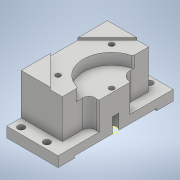
# Autodesk Inventor part: FAB-OX0001
Saved by Autodesk Inventor 2020 (Build 240168000, 168)
## iProperties
Created: 2017-01-19
Part Number: FAB-OX0001
Material: Generic
Document SubType Name: Modeling
Designer: map
Density: 1 g/cm^3
Appearance: Default
Author: map
Revision Number: 01
Autodesk Inventor part; units mm, degrees
ref_plane "YZ Plane" through (0, 0, 0) normal (1, 0, 0) x (0, 1, 0)
ref_plane "XZ Plane" through (0, 0, 0) normal (0, 1, 0) x (-1, 0, 0)
derived "FAB-P0038 - BS2 Optics Mount.ipt"
sketch "EXPORTED" plane through (-45, 40, 0) normal (0, 0, -1) x (-1, 0, 0)
  circle A0 centre (-33, -90) radius 3.3
  circle A1 centre (-8, -90) radius 3.3
  circle A2 centre (-19.9813, -66.0965) radius 4
  circle A3 centre (-46.0778, -40) radius 4
  circle A4 centre (-19.9813, -13.9035) radius 4
  circle A5 centre (-33, 10) radius 3.3
  circle A6 centre (-8, 10) radius 3.3
  circle A7 centre (-20.5, 10) radius 2
  line L0 (-5.7006, -21) -> (-19.7006, -7)
  line L1 (-19.7006, -73) -> (-5.7006, -59)
  line L2 (0, -97) -> (-50.5, -97)
  line L3 (-50.5, -97) -> (-50.5, -80)
  line L4 (0, -80) -> (0, -97)
  line L5 (0, 17) -> (0, 0)
  line L6 (-50.5, 17) -> (0, 17)
  line L7 (-50.5, 0) -> (-50.5, 17)
  point P0 (-45, -40)
ref_plane "LensMountFoot" through (-25.2994, 33, 47.902) normal (0, 0, 1) x (1, 0, 0)
ref_plane "GoniometerFoot" through (-11, -6, 37) normal (0, 0, 1) x (1, 0, 0)
ref_plane "Table" through (-45, 40, 0) normal (0, 0, -1) x (-1, 0, 0)
sketch "Sketch8" plane through (-45, 40, 0) normal (0, 0, -1) x (-1, 0, 0)
  line L0 (0, -96) -> (-50.5, -96)
  line L1 (-50.5, -96) -> (-50.5, 16)
  line L2 (-50.5, 16) -> (0, 16)
  line L3 (0, 16) -> (0, -96)
  line L4 (0, -80) -> (0, -97) projected
  line L5 (-50.5, -97) -> (-50.5, -80) projected
  circle A0 centre (-8, -90) radius 3.3 construction
  circle A1 centre (-8, 10) radius 3.3 construction
  line L6 (0, -40) -> (-50.5, -40) construction
  line L7 (-8, -90) -> (-8, 10) construction
  point P0 (-45, -40)
  point P1 (-8, -40)
  dimension "d15" = 112
  constraints: 12 end point, 3 midpoint, 2 collinear, 2 parallel, 1 horizontal, 1 perpendicular, 1 point on line, 1 vertical
  measures "d15" distance of L0.end L1.end
extrude "Bulk" add sketch "Sketch8" against normal up to surface (47.902 mm away)
ref_plane "Work Plane7" through (-45, 40, 10) normal (0, 0, -1) x (-1, 0, 0)
sketch "Sketch11" plane through (-45, 40, 10) normal (0, 0, -1) x (-1, 0, 0)
  circle A0 centre (-33, -90) radius 3.3 construction
  circle A1 centre (-8, -90) radius 3.3 construction
  circle A2 centre (-33, 10) radius 3.3 construction
  circle A3 centre (-8, 10) radius 3.3 construction
  line L0 (-50.5, -96) -> (-50.5, 16) construction
  line L1 (0, 16) -> (0, -96) construction
  line L2 (-50.5, -96) -> (0, -96)
  line L3 (0, -96) -> (0, -82)
  line L4 (0, -82) -> (-50.5, -82)
  line L5 (-50.5, -82) -> (-50.5, -96)
  line L6 (-50.5, 2) -> (0, 2)
  line L7 (0, 2) -> (0, 16)
  line L8 (0, 16) -> (-50.5, 16)
  line L9 (-50.5, 16) -> (-50.5, 2)
  line L10 (-50.5, -96) -> (0, -96) construction
  point P0 (-45, -40)
  point P1 (0, -89)
  dimension "d38" = 8
  constraints: 16 end point, 4 parallel, 3 point on line, 2 horizontal, 2 perpendicular, 1 collinear, 1 midpoint
  measures "d38" distance from line of L4 A0.centre
extrude "Feet" cut sketch "Sketch11" against normal through all
sketch "AlignmentFeatures" plane through (-45, 40, 0) normal (0, 0, -1) x (-1, 0, 0)
  line L0 (-19.9813, 10) -> (-19.9813, -90) construction
  line L1 (-19.9813, -92.5) -> (-19.9813, -87.5) construction
  line L2 (-17.9813, -92.5) -> (-17.9813, -87.5)
  line L3 (-21.9813, -87.5) -> (-21.9813, -92.5)
  arc A0 (-21.9813, -92.5) -> (-17.9813, -92.5) centre (-19.9813, -92.5) ccw
  arc A1 (-17.9813, -87.5) -> (-21.9813, -87.5) centre (-19.9813, -87.5) ccw
  line L4 (-50.5, 16) -> (0, 16) construction
  line L5 (0, -96) -> (-50.5, -96) construction
  point P0 (-45, -40)
  point P1 (-33, -90)
  point P2 (-8, -90)
  point P3 (-19.9813, -66.0965)
  point P4 (-19.9813, -13.9035)
  point P5 (-8, 10)
  point P6 (-33, 10)
  dimension "d108" = 2.5
  dimension "d109" = 4
  dimension "d120" = 6
  dimension "d121" = 6
  constraints: 10 end point, 4 point on circle, 4 tangent, 3 point on line, 2 centre point, 2 coincident, 1 midpoint, 1 parallel
  measures "d108" distance of L0.end L1.end
  measures "d109" diameter of A1
  measures "d120" distance from line of L4 L0.start
  measures "d121" distance from line of L5 L0.end
hole "AlignmentPostHoles" at (-25.0187, 50, 0) at (-25.0187, -52.5, 0) at (-25.0187, -47.5, 0) direction (0, 0, 1) diameter 4 depth 9
extrude "AlignmentSlot" cut sketch "AlignmentFeatures" against normal up to surface (9 mm away)
sketch "Sketch14" plane through (-45, 40, 0) normal (0, 0, -1) x (-1, 0, 0)
  line L0 (-50.5, -96) -> (-50.5, 16) projected
  line L1 (-50.5, -80) -> (0, -80)
  line L2 (0, -80) -> (0, 0)
  line L3 (0, 0) -> (-50.5, 0)
  line L4 (-50.5, 0) -> (-50.5, -80)
  line L5 (0, 16) -> (0, -96) projected
  point P0 (-45, -40)
  point P1 (-50.5, -40)
  dimension "d39" = 80
  constraints: 8 end point, 2 midpoint, 2 parallel, 1 collinear, 1 horizontal, 1 perpendicular, 1 point on line
  measures "d39" distance between parallel lines of L3 L1
extrude "FootRecess" cut sketch "Sketch14" against normal blind 2
sketch "Sketch12" plane through (-45, -42, 47.902) normal (0, 0, 1) x (1, 0, 0)
  line L0 (5.7006, 61) -> (19.7006, 75) construction
  line L1 (19.7006, 9) -> (5.7006, 23) construction
  line L2 (28.7006, 0) -> (0, 0)
  line L3 (0, 0) -> (0, 28.7006)
  line L4 (0, 28.7006) -> (28.7006, 0)
  line L5 (0, 0) -> (0, 84) projected
  line L6 (0, 0) -> (50.5, 0) projected
  line L7 (0, 55.2994) -> (0, 84)
  line L8 (0, 84) -> (28.7006, 84)
  line L9 (28.7006, 84) -> (0, 55.2994)
  line L10 (50.5, 84) -> (0, 84) projected
  point P0 (45, 42)
  point P1 (19.9813, 15.9035)
  point P2 (19.9813, 68.0965)
  constraints: 12 end point, 6 collinear
extrude "LensMountAlignmentFeatures" add sketch "Sketch12" along normal blind 2.1
sketch "Sketch13" plane through (-45, -42, 50.002) normal (0, 0, 1) x (1, 0, 0)
  line L0 (0, 84) -> (50.5, 84) projected
  line L1 (0, 0) -> (50.5, 0) projected
  line L2 (50.5, 84) -> (40.0778, 84)
  line L3 (40.0778, 84) -> (40.0778, 0)
  line L4 (40.0778, 0) -> (50.5, 0)
  line L5 (50.5, 0) -> (50.5, 84)
  line L6 (19.7006, 9) -> (5.7006, 23) projected
  line L7 (0, 28.7006) -> (28.7006, 0) projected
  line L8 (28.7006, 0) -> (50.5, 0) projected
  line L9 (50.5, 84) -> (50.5, 0) projected
  line L10 (50.5, 84) -> (28.7006, 84) projected
  line L11 (28.7006, 84) -> (0, 55.2994) projected
  line L12 (0, 28.7006) -> (0, 55.2994) projected
  line L13 (16.3892, 12.3114) -> (24.8745, 20.7967) construction
  line L14 (28.7006, 0) -> (0, 28.7006) construction
  line L15 (20.6318, 25.0393) -> (29.1171, 16.5541)
  circle A0 centre (46.0778, 42) radius 27.5
  point P0 (45, 42)
  point P1 (19.9813, 15.9035)
  dimension "d28" = 12
  dimension "d56" = 12
  dimension "d57" = 55
  dimension "d73" = 6
  constraints: 12 end point, 3 perpendicular, 3 point on line, 2 parallel, 1 centre point, 1 coincident, 1 horizontal, 1 midpoint
  measures "d28" distance of L13.end L13.start
  measures "d56" distance of L15.start L15.end
  measures "d57" diameter of A0
  measures "d73" distance from line of L3 A0.centre
extrude "GoniometerCutout" cut sketch "Sketch13" against normal up to surface (13.002 mm away) contours L0 L5 A0 L3 | A0 L5 L3 | L3 A0 | A0 L5 | A0 L5 L1 L3
hole "TableBoltHoles" at (-12, -50, 0) at (-37, -50, 0) at (-37, 50, 0) at (-12, 50, 0) direction (0, 0, 1) diameter 6.6 end through all clearance for "Socket Head Cap Screw ISO 4762" size "M6" standard "ISO"
sketch "Sketch15" plane through (-45, 40, 2) normal (0, 0, -1) x (-1, 0, 0)
  circle A0 centre (-46.0778, -40) radius 4 projected
  circle A1 centre (-19.9813, -66.0965) radius 4 projected
  circle A2 centre (-19.9813, -13.9035) radius 4 projected
  point P0 (-45, -40)
hole "LensMountBoltHoles" at (-25.0187, -26.0965, 2) at (-25.0187, 26.0965, 2) direction (0, 0, 1) diameter 5 end through all counterbore diameter 10 counterbore depth 25.5
sketch "Sketch17" plane through (-4.9222, 42, 37) normal (0, 0, 1) x (1, 0, 0)
  line L0 (6, -90.0117) -> (6, -64) construction
  line L1 (12, -90.0117) -> (12, -64)
  line L2 (0, -64) -> (0, -90.0117)
  arc A0 (0, -90.0117) -> (12, -90.0117) centre (6, -90.0117) ccw
  arc A1 (12, -64) -> (0, -64) centre (6, -64) ccw
  line L3 (0, -84) -> (0, -68.8375) projected
  line L4 (9.5, -18) -> (9.5, 9.0033) construction
  line L5 (19, -18) -> (19, 9.0033)
  line L6 (0, 9.0033) -> (0, -18)
  arc A2 (0, -18) -> (19, -18) centre (9.5, -18) ccw
  arc A3 (19, 9.0033) -> (0, 9.0033) centre (9.5, 9.0033) ccw
  line L7 (0, -15.1625) -> (0, 0) projected
  point P0 (6, -77.0058)
  point P1 (6, -42)
  point P2 (9.5, -4.4984)
  point P3 (6, -42)
  dimension "d85" = 12
  dimension "d89" = 22
  dimension "d93" = 19
  dimension "d94" = 24
  constraints: 16 end point, 8 point on circle, 8 tangent, 4 centre point, 2 collinear, 2 midpoint, 2 parallel, 2 vertical, 1 coincident
  measures "d85" diameter of A1
  measures "d89" distance of L0.end point (6, -42)
  measures "d93" diameter of A2
  measures "d94" vertical distance of point (6, -42) L4.start
extrude "Extrusion13" cut sketch "Sketch17" against normal up to surface (27 mm away)
fillet "Fillet5" radius 2 4 edges at (5.5, -17.9449, 23.5) (5.5, 14.5449, 23.5) (-4.9222, -26.8375, 42.451) (-4.9222, 26.8375, 42.451)
sketch "Sketch21" plane through (-45, 40, 0) normal (0, 0, -1) x (-1, 0, 0)
  line L0 (0, -96) -> (-50.5, -96) projected
  line L1 (0, 16) -> (-50.5, 16) projected
  line L2 (-50.5, -96) -> (-50, -96)
  line L3 (-50, -96) -> (-50, 16)
  line L4 (-50, 16) -> (-50.5, 16)
  line L5 (-50.5, 16) -> (-50.5, -96)
  point P0 (-45, -40)
  dimension "d122" = 0.5
  constraints: 8 end point, 2 parallel, 1 horizontal, 1 perpendicular, 1 point on line
  measures "d122" distance of L4.end L3.end
extrude "Extrusion15" cut sketch "Sketch21" against normal through all
hole "GoniometerBoltHole" at (1.0778, 0, 2) direction (0, 0, 1) diameter 5 end through all counterbore diameter 10 counterbore depth 14.5
equation "\"d56\" = d28"
body "Solid2"
